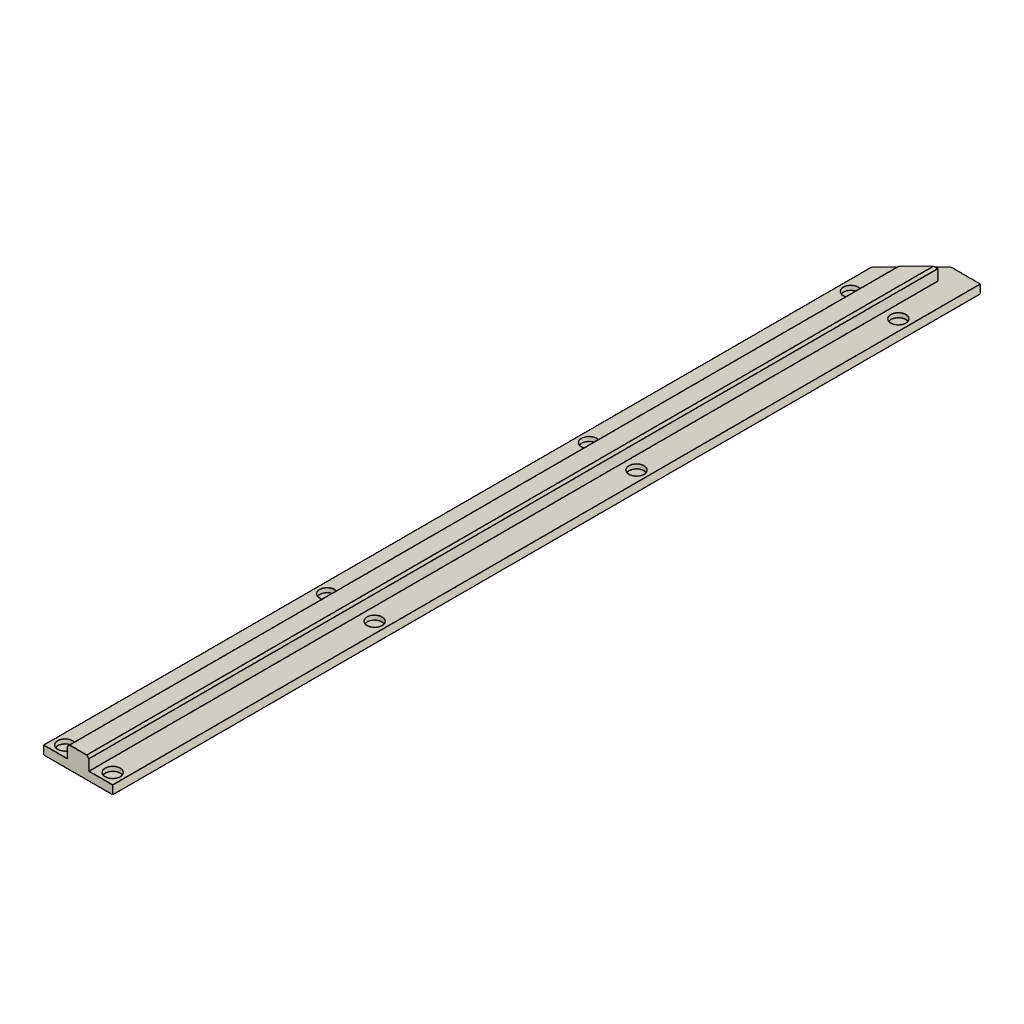
arcade_buttons_conduit (Autodesk Fusion 360 archive; units mm, degrees)
design "Arcade Buttons Conduit Top"
part number: 2026-09-19-15-15-46-900
Autodesk Fusion 360 part; units mm, degrees
note: some values were not read from the file. Set by a fixed rule: which sketch regions a step uses.
sketch "3D-printed conduit top outline" plane through (0, 0, 0) normal (0, 1, 0) x (1, 0, 0)
  line L0 (0, 0) -> (16, 0)
  line L1 (16, 0) -> (16, -2)
  line L2 (16, -2) -> (0, -2)
  line L3 (0, -2) -> (0, 0)
  dimension "d7" = 16
  dimension "d8" = 2
  constraint horizontal L0
  constraint vertical L1
  constraint horizontal L2
  constraint vertical L3
  constraint coincident L0.start L3.end
  measures "d7" distance of L0.start L0.end
  measures "d8" distance of L0.start L2.end
extrude "Extrude1" add sketch "3D-printed conduit top outline" along normal blind 201
sketch "Magnet holes" plane through (0, 0, 2) normal (0, 0, 1) x (-1, 0, 0)
  line L0 (0, 0) -> (-16, 0)
  line L1 (-16, 0) -> (-16, -201)
  line L2 (-16, -201) -> (0, -201)
  line L3 (0, -201) -> (0, 0)
  circle A0 centre (-2.5, -2.5) radius 2.5
  circle A1 centre (-13.5, -2.5) radius 2.5
  circle A2 centre (-2.5, -2.5) radius 1.75
  circle A3 centre (-13.5, -2.5) radius 1.75
  circle A4 centre (-2.5, -63.1667) radius 1.75
  circle A5 centre (-2.5, -63.1667) radius 2.5
  circle A6 centre (-13.5, -63.1667) radius 2.5
  circle A7 centre (-13.5, -63.1667) radius 1.75
  circle A8 centre (-2.5, -123.8333) radius 1.75
  circle A9 centre (-2.5, -123.8333) radius 2.5
  circle A10 centre (-13.5, -123.8333) radius 2.5
  circle A11 centre (-13.5, -123.8333) radius 1.75
  circle A12 centre (-2.5, -184.5) radius 1.75
  circle A13 centre (-2.5, -184.5) radius 2.5
  circle A14 centre (-13.5, -184.5) radius 2.5
  circle A15 centre (-13.5, -184.5) radius 1.75
  dimension "d11" = 5
  dimension "d12" = 5
  dimension "d13" = 3.5
  dimension "d14" = 3.5
  dimension "d17" = 0
  dimension "d18" = -182
  constraint concentric A0 A2
  constraint concentric A1 A3
  constraint tangent L3 A0
  constraint tangent L0 A0
  constraint tangent L1 A1
  constraint tangent L0 A1
  measures "d11" diameter of A0
  measures "d12" diameter of A1
  measures "d13" diameter of A2
  measures "d14" diameter of A3
extrude "Extrude2" cut sketch "Magnet holes" against normal blind 1 contours A2 | A3 | A4 | A7 | A8 | A11 | A12 | A15
sketch "Support rib" plane through (0, 0, 2) normal (0, 0, 1) x (-1, 0, 0)
  line L0 (0, 0) -> (-16, 0)
  line L1 (-16, 0) -> (-16, -201)
  line L2 (-16, -201) -> (0, -201)
  line L3 (0, -201) -> (0, 0)
  circle A0 centre (-13.5, -184.5) radius 1.75
  circle A1 centre (-13.5, -63.1667) radius 1.75
  circle A2 centre (-2.5, -2.5) radius 1.75
  circle A3 centre (-2.5, -123.8333) radius 1.75
  circle A4 centre (-2.5, -184.5) radius 1.75
  circle A5 centre (-2.5, -63.1667) radius 1.75
  circle A6 centre (-13.5, -2.5) radius 1.75
  circle A7 centre (-13.5, -123.8333) radius 1.75
  line L4 (-5.5, 0) -> (-10.5, 0)
  line L5 (-10.5, 0) -> (-10.5, -201)
  line L6 (-10.5, -201) -> (-5.5, -201)
  line L7 (-5.5, -201) -> (-5.5, 0)
  dimension "d23" = 5
  dimension "d24" = 5.5
  dimension "d25" = 5.5
  constraint horizontal L4
  constraint vertical L5
  constraint horizontal L6
  constraint vertical L7
  constraint coincident L2 L5.end
  constraint coincident L0 L4.start
  measures "d23" distance of L5 L7
  measures "d24" distance of L3 L7
  measures "d25" distance of L1 L5
extrude "Extrude3" add sketch "Support rib" along normal blind 3 contours L0 L2 L4 L5 L6 L7
chamfer "Chamfer1" distance 0.5 angle 45 2 edges at (5.5, 100.5, 5) (10.5, 100.5, 5)
sketch "End chamfer" plane through (0, 0, 2) normal (0, 0, 1) x (-1, 0, 0)
  line L0 (-10.5, -201) -> (-10.5, 0)
  line L1 (-10.5, 0) -> (-16, 0)
  line L2 (-16, 0) -> (-16, -201)
  line L3 (-16, -201) -> (-10.5, -201)
  circle A0 centre (-13.5, -123.8333) radius 1.75
  circle A1 centre (-13.5, -2.5) radius 1.75
  circle A2 centre (-13.5, -63.1667) radius 1.75
  circle A3 centre (-13.5, -184.5) radius 1.75
  line L4 (0, -191.828) -> (-9.172, -201)
  line L5 (0, 0) -> (0, -201)
  line L6 (-14.8289, -201) -> (0, -186.1711)
  line L7 (0, -191.828) -> (0, -201)
  line L8 (0, -201) -> (-9.172, -201)
  line L9 (-9.172, -201) -> (-14.8289, -201)
  line L10 (0, -191.828) -> (0, -186.1711)
  dimension "d30" = 6.828
  dimension "d31" = 135
  dimension "d32" = 4
  constraint coincident L3 L4.end
  constraint coincident L4.start L5
  constraint coincident L3 L6.start
  constraint coincident L5 L6.end
  constraint parallel L4 L6
  constraint coincident L5.end L7.end
  measures "d30" distance of L2.end L4.end
  measures "d31" angle of L3 L4
  measures "d32" distance of L4 L6
extrude "Extrude4" cut sketch "End chamfer" along normal blind 3 and the other way blind 2 contours L4 L5 L7 L8
extrude "Extrude5" cut sketch "End chamfer" along normal blind 3 contours L0 L3 L6 L9 | L0 L4 L5 L6 L9 L10
equation "conduit_length = 201 mm"
equation "conduit_width = 16 mm"
equation "conduit_wall_thickness = 2 mm"
equation "magnet_diameter = 3 mm"
equation "magnet_height = 1 mm"
equation "number_of_magnets_on_a_side = 4"
equation "d7 = conduit_width"
equation "d8 = conduit_wall_thickness"
equation "d9 = conduit_length"
equation "d11 = magnet_diameter + 2 mm"
equation "d12 = magnet_diameter + 2 mm"
equation "d13 = magnet_diameter + 0.5 mm"
equation "d14 = magnet_diameter + 0.5 mm"
equation "d16 = number_of_magnets_on_a_side"
equation "d18 = -conduit_length + ( magnet_diameter + 2 mm ) + 14 mm"
equation "d19 = -magnet_height"
equation "rib_width = 5 mm"
equation "rib_height = 3 mm"
equation "d23 = rib_width"
equation "d24 = ( conduit_width - rib_width ) / 2"
equation "d26 = rib_height"
equation "rib_chamfer = 0.5 mm"
equation "d29 = rib_chamfer"
equation "d32 = 2 * conduit_wall_thickness"
equation "d33 = rib_height"
equation "d35 = conduit_wall_thickness"
equation "d37 = rib_height"
named bodies: "Arcade buttons conduit top"

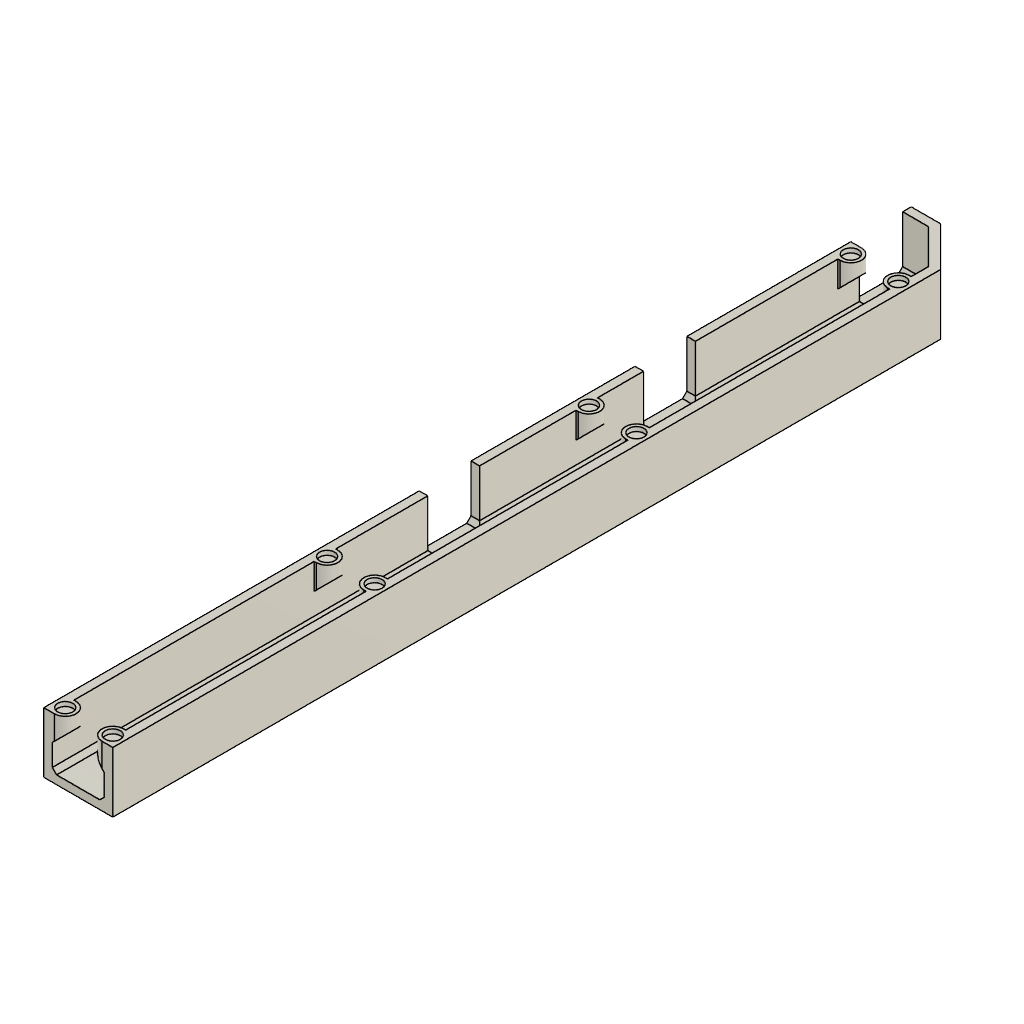
design "Arcade Buttons Conduit Bottom"
part number: 2026-09-19-14-55-36-645
Autodesk Fusion 360 part; units mm, degrees
sketch "3D-printed conduit outline" plane through (0, 0, 0) normal (0, 1, 0) x (1, 0, 0)
  line L0 (0, 0) -> (16, 0)
  line L1 (16, 0) -> (16, -14)
  line L2 (16, -14) -> (0, -14)
  line L3 (0, -14) -> (0, 0)
  line L4 (2, -14) -> (14, -14)
  line L5 (14, -14) -> (14, -2)
  line L6 (14, -2) -> (2, -2)
  line L7 (2, -2) -> (2, -14)
  dimension "d8" = 14
  dimension "d9" = 16
  dimension "d10" = 2
  dimension "d11" = 2
  dimension "d12" = 2
  constraint horizontal L0
  constraint vertical L1
  constraint horizontal L2
  constraint vertical L3
  constraint coincident L0.start L3.end
  constraint horizontal L4
  constraint vertical L5
  constraint horizontal L6
  constraint vertical L7
  constraint coincident L2 L4.start
  measures "d8" distance of L0.start L2.end
  measures "d9" distance of L0.start L0.end
  measures "d10" distance of L1 L5
  measures "d11" distance of L3 L7
  measures "d12" distance of L0 L6
extrude "Extrude1" add sketch "3D-printed conduit outline" along normal blind 201 contours L0 L1 L2 L3 L5 L6 L7
sketch "Magnet holders" plane through (0, 0, 14) normal (0, 0, 1) x (-1, 0, 0)
  line L0 (0, 0) -> (-2, 0)
  line L1 (-2, 0) -> (-2, -201)
  line L2 (-2, -201) -> (0, -201)
  line L3 (0, -201) -> (0, 0)
  line L4 (-14, 0) -> (-16, 0)
  line L5 (-16, 0) -> (-16, -201)
  line L6 (-16, -201) -> (-14, -201)
  line L7 (-14, -201) -> (-14, 0)
  circle A0 centre (-2.5, -2.5) radius 2.5
  circle A1 centre (-2.5, -2.5) radius 1.75
  line L8 (-14, 0) -> (-2, 0)
  line L9 (0, 0) -> (-2.5, 0)
  line L10 (-2.5, 0) -> (-2.5, -5)
  line L11 (-2.5, -5) -> (0, -5)
  line L12 (0, -5) -> (0, 0)
  circle A2 centre (-13.5, -2.5) radius 2.5
  circle A3 centre (-13.5, -2.5) radius 1.75
  line L13 (-16, 0) -> (-13.5, 0)
  line L14 (-13.5, 0) -> (-13.5, -5)
  line L15 (-13.5, -5) -> (-16, -5)
  line L16 (-16, -5) -> (-16, 0)
  circle A4 centre (-2.5, -63.1667) radius 1.75
  circle A5 centre (-2.5, -63.1667) radius 2.5
  line L17 (-2.5, -60.6667) -> (-2.5, -65.6667)
  line L18 (-2.5, -65.6667) -> (0, -65.6667)
  line L19 (0, -65.6667) -> (0, -60.6667)
  line L20 (0, -60.6667) -> (-2.5, -60.6667)
  circle A6 centre (-13.5, -63.1667) radius 1.75
  circle A7 centre (-13.5, -63.1667) radius 2.5
  line L21 (-13.5, -60.6667) -> (-13.5, -65.6667)
  line L22 (-13.5, -65.6667) -> (-16, -65.6667)
  line L23 (-16, -65.6667) -> (-16, -60.6667)
  line L24 (-16, -60.6667) -> (-13.5, -60.6667)
  circle A8 centre (-2.5, -123.8333) radius 1.75
  circle A9 centre (-2.5, -123.8333) radius 2.5
  line L25 (-2.5, -121.3333) -> (-2.5, -126.3333)
  line L26 (-2.5, -126.3333) -> (0, -126.3333)
  line L27 (0, -126.3333) -> (0, -121.3333)
  line L28 (0, -121.3333) -> (-2.5, -121.3333)
  circle A10 centre (-13.5, -123.8333) radius 1.75
  circle A11 centre (-13.5, -123.8333) radius 2.5
  line L29 (-13.5, -121.3333) -> (-13.5, -126.3333)
  line L30 (-13.5, -126.3333) -> (-16, -126.3333)
  line L31 (-16, -126.3333) -> (-16, -121.3333)
  line L32 (-16, -121.3333) -> (-13.5, -121.3333)
  circle A12 centre (-2.5, -184.5) radius 1.75
  circle A13 centre (-2.5, -184.5) radius 2.5
  line L33 (-2.5, -182) -> (-2.5, -187)
  line L34 (-2.5, -187) -> (0, -187)
  line L35 (0, -187) -> (0, -182)
  line L36 (0, -182) -> (-2.5, -182)
  circle A14 centre (-13.5, -184.5) radius 1.75
  circle A15 centre (-13.5, -184.5) radius 2.5
  line L37 (-13.5, -182) -> (-13.5, -187)
  line L38 (-13.5, -187) -> (-16, -187)
  line L39 (-16, -187) -> (-16, -182)
  line L40 (-16, -182) -> (-13.5, -182)
  dimension "d15" = 5
  dimension "d16" = 3.5
  dimension "d17" = 5
  dimension "d18" = 3.5
  dimension "d21" = 0
  dimension "d22" = -182
  constraint concentric A0 A1
  constraint tangent A0 L8
  constraint tangent L3 A0
  constraint horizontal L9
  constraint vertical L10
  constraint horizontal L11
  constraint vertical L12
  constraint coincident L0.start L3.end
  constraint tangent A0 L11
  constraint coincident A0 L9.end
  constraint concentric A2 A3
  constraint tangent L5 A2
  constraint tangent L8 A2
  constraint horizontal L13
  constraint vertical L14
  constraint horizontal L15
  constraint vertical L16
  constraint coincident L4.end L5.start
  constraint tangent A2 L15
  constraint coincident A2 L13.end
  measures "d15" diameter of A0
  measures "d16" diameter of A1
  measures "d17" diameter of A2
  measures "d18" diameter of A3
sketch "End wall" plane through (0, 201, 0) normal (0, 1, 0) x (-1, 0, 0)
  line L0 (-2, 2) -> (-14, 2)
  line L1 (-14, 2) -> (-14, 14)
  line L2 (-14, 14) -> (-16, 14)
  line L3 (-16, 14) -> (-16, 0)
  line L4 (-16, 0) -> (0, 0)
  line L5 (0, 0) -> (0, 14)
  line L6 (0, 14) -> (-2, 14)
  line L7 (-2, 14) -> (-2, 2)
  line L8 (-16, 0) -> (0, 0)
  line L9 (0, 0) -> (0, 14)
  line L10 (0, 14) -> (-16, 14)
  line L11 (-16, 14) -> (-16, 0)
  constraint horizontal L8
  constraint vertical L9
  constraint horizontal L10
  constraint vertical L11
  constraint coincident L5.end L6.start
  constraint coincident L3.end L4.start
extrude "Extrude5" add sketch "End wall" against normal blind 2
extrude "Extrude2" add sketch "Magnet holders" against normal blind 3 contours L1 A0 L8 L9 | L1 A0 A1 L10 | A0 A1 L10 | L1 A0 A1 L10 | L1 A0 L11 | L1 A1 L10 | A1 L10 | L1 A5 L20 | L1 A4 A5 L17 | L1 A4 A5 L17 | L1 A5 L18 | A4 A5 L17 | L1 A4 L17 | A4 L17 | L1 A9 L28 | L1 A8 A9 L25 | L1 A8 A9 L25 | L1 A9 L26 | A8 A9 L25 | L1 A8 L25 | A8 L25 | L1 A13 L36 | L1 A12 A13 L33 | L1 A12 A13 L33 | L1 A13 L34 | A12 A13 L33 | L1 A12 L33 | A12 L33 | L7 L8 A2 L13 | L7 A2 A3 L14 | A2 A3 L14 | L7 A3 L14 | A3 L14 | L7 A2 L15 | L7 A2 A3 L14 | L7 A7 L24 | L7 A6 A7 L21 | L7 A7 L22 | L7 A6 A7 L21 | A6 A7 L21 | L7 A6 L21 | A6 L21 | L7 A11 L32 | L7 A10 A11 L29 | L7 A11 L30 | L7 A10 A11 L29 | A10 A11 L29 | L7 A10 L29 | A10 L29 | L7 A15 L40 | L7 A14 A15 L37 | L7 A15 L38 | L7 A14 A15 L37 | A14 A15 L37 | L7 A14 L37 | A14 L37
extrude "Extrude6" cut sketch "Magnet holders" against normal blind 1 contours L1 A1 | L1 A1 L10 | A1 L10 | L1 A4 | L1 A4 L17 | A4 L17 | L1 A8 | L1 A8 L25 | A8 L25 | L1 A12 | L1 A12 L33 | A12 L33 | L7 A3 L14 | L7 A3 | A3 L14 | L7 A6 L21 | L7 A6 | A6 L21 | L7 A10 L29 | L7 A10 | A10 L29 | L7 A14 L37 | L7 A14 | A14 L37
chamfer "Chamfer2" distance 2.9999 angle 45 11 edges at (2, 2.5, 11) (2, 63.1667, 11) (2, 123.8333, 11) (2, 2.5, 11) (2, 123.8333, 11) (2, 63.1667, 11) (2, 184.5, 11) (14, 2.5, 11) (14, 63.1667, 11) (14, 123.8333, 11) (14, 184.5, 11)
sketch "Arcade button outlets" plane through (0, 0, 0) normal (-1, 0, 0) x (0, -1, 0)
  line L0 (0, 0) -> (0, 14)
  line L1 (0, 14) -> (-201, 14)
  line L2 (-201, 14) -> (-201, 0)
  line L3 (-201, 0) -> (0, 0)
  line L4 (-199, 14) -> (-187, 14)
  line L5 (-187, 14) -> (-187, 2)
  line L6 (-187, 2) -> (-199, 2)
  line L7 (-199, 2) -> (-199, 14)
  line L8 (-149, 14) -> (-137, 14)
  line L9 (-137, 14) -> (-137, 2)
  line L10 (-137, 2) -> (-149, 2)
  line L11 (-149, 2) -> (-149, 14)
  line L12 (-99, 14) -> (-87, 14)
  line L13 (-87, 14) -> (-87, 2)
  line L14 (-87, 2) -> (-99, 2)
  line L15 (-99, 2) -> (-99, 14)
  dimension "d29" = 2
  dimension "d30" = 12
  dimension "d31" = 12
  dimension "d32" = 12
  dimension "d33" = 2
  dimension "d34" = 38
  dimension "d35" = 38
  constraint horizontal L4
  constraint vertical L5
  constraint horizontal L6
  constraint vertical L7
  constraint coincident L1 L4.start
  constraint horizontal L8
  constraint vertical L9
  constraint horizontal L10
  constraint vertical L11
  constraint coincident L1 L8.start
  constraint horizontal L12
  constraint vertical L13
  constraint horizontal L14
  constraint vertical L15
  constraint coincident L1 L12.start
  constraint collinear L6 L10
  constraint collinear L10 L14
  measures "d29" distance of L3 L6
  measures "d30" distance of L5.end L6.end
  measures "d31" distance of L9.end L10.end
  measures "d32" distance of L13.end L14.end
  measures "d33" distance of L2 L7
  measures "d34" distance of L5 L11
  measures "d35" distance of L9 L15
extrude "Extrude4" cut sketch "Arcade button outlets" against normal blind 2 contours L1 L12 L13 L14 L15 | L1 L4 L5 L6 L7 | L1 L8 L9 L10 L11
sketch "End chamfer" plane through (0, 0, 14) normal (0, 0, 1) x (-1, 0, 0)
  line L0 (0, -199) -> (-14, -199)
  line L1 (-14, -199) -> (-14, -187)
  line L2 (-14, -187) -> (-13.5, -187)
  arc A0 (-13.5, -187) -> (-13.5, -182) centre (-13.5, -184.5) ccw
  line L3 (-13.5, -182) -> (-14, -182)
  line L4 (-14, -182) -> (-14, -126.3333)
  line L5 (-14, -126.3333) -> (-13.5, -126.3333)
  arc A1 (-13.5, -126.3333) -> (-13.5, -121.3333) centre (-13.5, -123.8333) ccw
  line L6 (-13.5, -121.3333) -> (-14, -121.3333)
  line L7 (-14, -121.3333) -> (-14, -65.6667)
  line L8 (-14, -65.6667) -> (-13.5, -65.6667)
  arc A2 (-13.5, -65.6667) -> (-13.5, -60.6667) centre (-13.5, -63.1667) ccw
  line L9 (-13.5, -60.6667) -> (-14, -60.6667)
  line L10 (-14, -60.6667) -> (-14, -5)
  line L11 (-14, -5) -> (-13.5, -5)
  arc A3 (-13.5, -5) -> (-13.5, 0) centre (-13.5, -2.5) ccw
  line L12 (-13.5, 0) -> (-16, 0)
  line L13 (-16, 0) -> (-16, -201)
  line L14 (-16, -201) -> (0, -201)
  line L15 (0, -201) -> (0, -199)
  circle A4 centre (-13.5, -2.5) radius 1.75
  circle A5 centre (-13.5, -63.1667) radius 1.75
  circle A6 centre (-13.5, -184.5) radius 1.75
  circle A7 centre (-13.5, -123.8333) radius 1.75
  line L16 (-6.8284, -201) -> (-16, -191.8284)
  line L17 (-4, -201) -> (-16, -189)
  line L18 (-2, -149) -> (-2, -182)
  line L19 (0, -193) -> (-8, -193)
  line L20 (0, -187) -> (0, -199)
  line L21 (-4, -193) -> (-8, -189)
  line L22 (-4, -193) -> (-0.3616, -193) construction
  line L23 (-8, -189) -> (-8, -193)
  line L24 (-10, -195) -> (-2, -187)
  line L25 (-2.5, -187) -> (0, -187)
  line L26 (-4, -201) -> (-6.8284, -201)
  line L27 (-16, -191.8284) -> (-16, -189)
  point P0 (-6, -191)
  dimension "d46" = 6
  dimension "d47" = 8
  dimension "d49" = 135
  dimension "d50" = 4
  dimension "d51" = 2
  dimension "d52" = 2
  constraint coincident L14 L16.start
  constraint coincident L13 L16.end
  constraint coincident L14 L17.start
  constraint horizontal L19
  constraint coincident L19.start L20
  constraint horizontal L22
  constraint coincident L19 L21.start
  constraint midpoint L19 L21.start
  constraint midpoint L24 P0
  constraint coincident L21 P0
  constraint coincident L24.end L25
  constraint perpendicular L21 L24
  constraint parallel L17 L21
  constraint parallel L16 L21
  constraint coincident L13 L17.end
  constraint coincident L17 L24.start
  measures "d46" distance of L0 L19
  measures "d47" distance of L19.start L19.end
  measures "d49" angle of L21 L22
  measures "d50" horizontal distance of L21.start L21.end
  measures "d51" distance of L20.start L24.end
  measures "d52" distance of L16 L17
extrude "Extrude8" add sketch "End chamfer" against normal blind 12 contours L0 L14 L16 L17 L26 | L0 L1 L16 L17 | L1 L13 L16 L17 L27
extrude "Extrude7" cut sketch "End chamfer" against normal blind 14 contours L0 L1 L13 L14 L16 | L0 L1 L16
chamfer "Chamfer4" distance 1 angle 45 11 edges at (2, 43.5, 2) (1, 87, 2) (1, 99, 2) (2, 118, 2) (1, 137, 2) (1, 149, 2) (2, 168, 2) (1, 187, 2) (3, 199, 2) (10, 195, 2) (14, 95.5, 2)
equation "conduit_length = 201 mm"
equation "conduit_width = 16 mm"
equation "conduit_height = 16 mm"
equation "conduit_wall_thickness = 2 mm"
equation "magnet_diameter = 3 mm"
equation "magnet_height = 1 mm"
equation "number_of_magnets_on_a_side = 4"
equation "d8 = conduit_height - conduit_wall_thickness"
equation "d9 = conduit_width"
equation "d10 = conduit_wall_thickness"
equation "d11 = conduit_wall_thickness"
equation "d12 = conduit_wall_thickness"
equation "d13 = conduit_length"
equation "d15 = magnet_diameter + 2 mm"
equation "d16 = magnet_diameter + 0.5 mm"
equation "d17 = magnet_diameter + 2 mm"
equation "d18 = magnet_diameter + 0.5 mm"
equation "d20 = number_of_magnets_on_a_side"
equation "d22 = -conduit_length + ( magnet_diameter + 2 mm ) + 14 mm"
equation "d23 = -( magnet_height + 2 mm )"
equation "d29 = conduit_wall_thickness"
equation "d33 = conduit_wall_thickness"
equation "d36 = -conduit_wall_thickness"
equation "d38 = -conduit_wall_thickness"
equation "d41 = -magnet_height"
equation "d47 = conduit_wall_thickness + ( conduit_width - 2 * conduit_wall_thickness ) / 2"
equation "d50 = ( conduit_wall_thickness + ( conduit_width - 2 * conduit_wall_thickness ) / 2 ) / 2"
equation "d51 = conduit_wall_thickness"
equation "d52 = conduit_wall_thickness"
equation "d53 = -( conduit_height - conduit_wall_thickness )"
equation "d55 = -( conduit_height - 2 * conduit_wall_thickness )"
named bodies: "Arcade buttons conduit bottom"

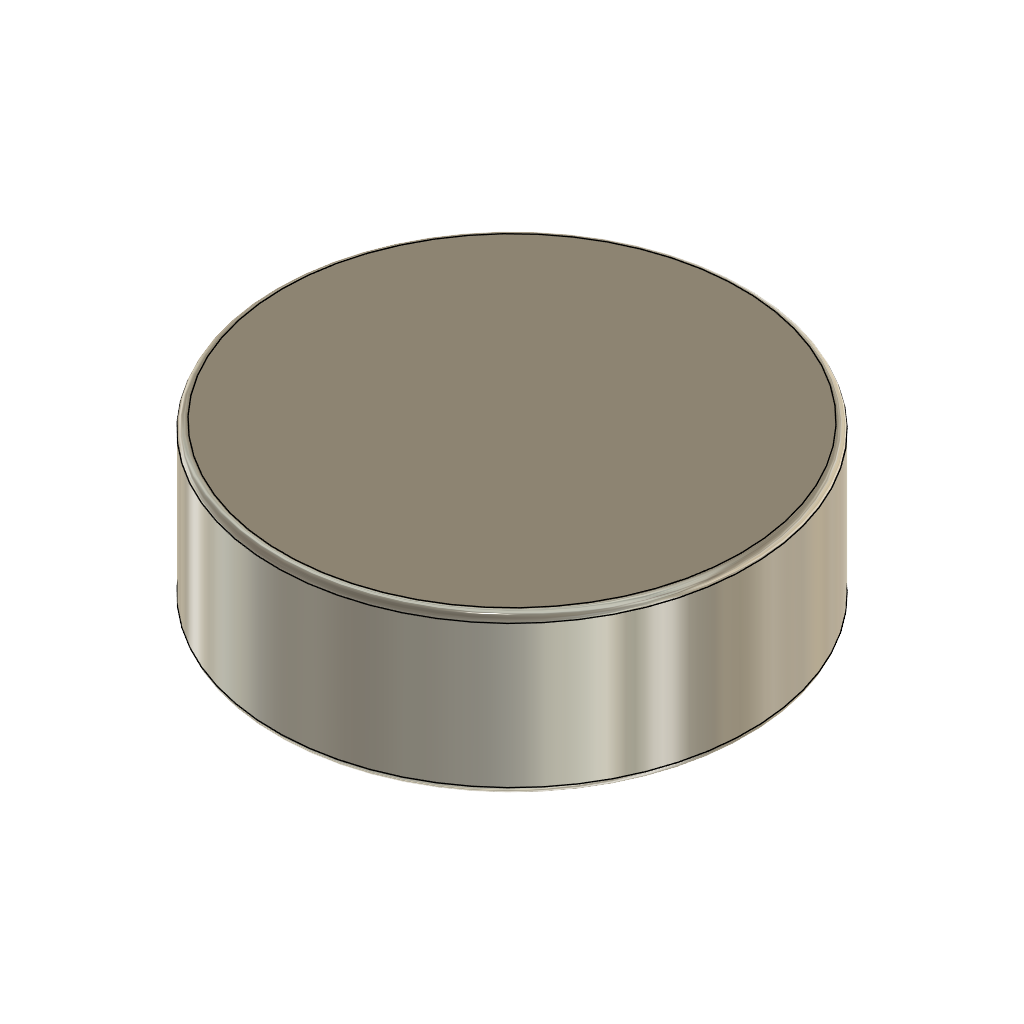
design "3 mm x 1 mm Neodymium Disc Magnet"
Autodesk Fusion 360 part; units mm, degrees
sketch "3 mm x 1 mm neodymium disc magnet" plane through (0, 0, 0) normal (0, 0, 1) x (1, 0, 0)
  circle A0 centre (0, 0) radius 1.5
  dimension "d1" = 3
  constraint coincident A0.centre origin
  measures "d1" diameter of A0
extrude "Extrude1" add sketch "3 mm x 1 mm neodymium disc magnet" along normal blind 1
fillet "Fillet1" radius 0.05 2 edges at (-1.3985, -0.5424, 1) (-1.3985, -0.5424, 0)
named bodies: "3 mm x 1 mm Neodymium Disc Magnet"
